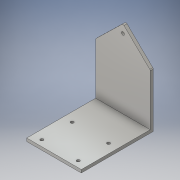
# Autodesk Inventor part: Braquet Rammasse-Balle
Saved by Autodesk Inventor 2016 (Build 200138000, 138)
## iProperties
Created: 2016-01-25
Part Number: Braquet Rammasse-Balle
Material: Generic
Document SubType Name: Modeling
Designer: ares-b02
Density: 1 g/cm^3
Appearance: Aluminum - Polished
Author: ares-b02
Autodesk Inventor part; units mm, degrees
ref_plane "YZ Plane" through (0, 0, 0) normal (1, 0, 0) x (0, 1, 0)
ref_plane "XZ Plane" through (0, 0, 0) normal (0, 1, 0) x (-1, 0, 0)
ref_plane "XY Plane" through (0, 0, 0) normal (0, 0, 1) x (1, 0, 0)
sketch "Sketch1" plane through (0, 0, 0) normal (0, 0, 1) x (1, 0, 0)
  line L0 (-48.8512, -88.9904) -> (65.4488, -88.9904)
  line L1 (65.4488, -88.9904) -> (65.4488, 23.9678)
  line L2 (64.4867, 26.2447) -> (10.5117, 78.7012)
  line L3 (6.086, 78.7012) -> (-47.889, 26.2447)
  line L4 (-48.8512, 23.9678) -> (-48.8512, -88.9904)
  circle A0 centre (8.2988, 63.4096) radius 3.175
  arc A1 (10.5117, 78.7012) -> (6.086, 78.7012) centre (8.2988, 76.4243) ccw
  arc A2 (-47.889, 26.2447) -> (-48.8512, 23.9678) centre (-45.6762, 23.9678) ccw
  arc A3 (65.4488, 23.9678) -> (64.4867, 26.2447) centre (62.2738, 23.9678) ccw
  point P0 (0, 0)
  point P1 (65.4488, 25.3096)
  point P2 (8.2988, 80.8517)
  point P3 (-48.8512, 25.3096)
  dimension "d0" = 114.3
  dimension "d1" = 114.3
  dimension "d2" = 114.3
  dimension "d3" = 57.15
  dimension "d4" = 6.35
  dimension "d5" = 152.4
  dimension "d6" = 3.175
  dimension "d29" = 57.15
  constraints: 10 end point, 6 point on circle, 6 point on line, 6 tangent, 4 centre point, 2 equal radius, 1 horizontal, 1 parallel, 1 perpendicular
  measures "d0" distance of L0.start L0.end
  measures "d1" distance of L0.end point (65.449, 25.31)
  measures "d2" distance of point (-48.851, 25.31) L0.start
  measures "d3" distance from line of L1 point (8.299, 80.852)
  measures "d4" diameter of A0
  measures "d5" distance from line of L0 A0.centre
  measures "d6" radius of A1
  measures "d29" distance from line of L1 A0.centre
extrude "Extrusion1" add sketch "Sketch1" against normal blind 6.35
sketch "Sketch2" plane through (0, 0, 0) normal (0, 0, 1) x (1, 0, 0)
  line L0 (65.4488, -88.9904) -> (-48.8512, -88.9904) projected
  line L1 (-48.8512, -88.9904) -> (65.4488, -88.9904)
  line L2 (65.4488, -88.9904) -> (65.4488, -82.6404)
  line L3 (65.4488, -82.6404) -> (-48.8512, -82.6404)
  line L4 (-48.8512, -82.6404) -> (-48.8512, -88.9904)
  point P0 (0, 0)
  dimension "d9" = 6.35
  dimension "d30" = 114.3
  constraints: 8 end point, 2 parallel, 1 horizontal, 1 perpendicular
  measures "d9" distance of L1.end L2.end
  measures "d30" distance of L2.end L3.end
extrude "Extrusion2" add sketch "Sketch2" along normal blind 144.4498
hole "Hole1" at (-29.8012, -82.6404, 131.7498) direction (0, -1, 0) diameter 6.35 end through all
pattern_linear "Rectangular Pattern1" count 2 spacing 63.5 along (0, 0, -1) count 2 spacing 76.2 along (1, 0, 0) of "Hole1"
body "Solid1"
